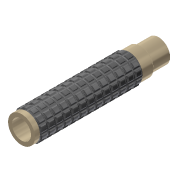
# Autodesk Inventor part: PP-10
Saved by Autodesk Inventor 2022 (Build 260148000, 148)
## iProperties
Created: 2008-09-23
Part Number: PP-10
Document SubType Name: Modeling
Designer: Mark Flayler
Mass: 8.28114 g
Surface Area: 19.0738 cm^2
Volume: 1.05358 cm^3
Density: 7.86 g/cm^3
Material: Steel, Mild
Description: GRIP
Appearance: Titanium - Polished
Author: Mark Flayler
Autodesk Inventor part; units mm, degrees
ref_plane "XZ Plane" through (0, 0, 0) normal (0, 1, 0) x (-1, 0, 0)
sketch "Sketch1" plane through (0, 0, 0) normal (0, 0, 1) x (1, 0, 0)
  line L0 (0, 0) -> (0, 40.8)
  line L1 (2.85, 0) -> (4, 0)
  line L2 (4, 0) -> (4, 35.25)
  line L3 (4, 35.25) -> (3.45, 35.8)
  line L4 (3.45, 35.8) -> (3.45, 40.8)
  line L5 (3.45, 40.8) -> (2.85, 40.8)
  line L6 (2.85, 40.8) -> (2.85, 0)
  dimension "d0" = 40.8
  dimension "d1" = 5.7
  dimension "d2" = 6.9
  dimension "d3" = 35.8
  dimension "d4" = 35.25
  dimension "d5" = 8
  constraints: 14 end point, 3 parallel, 2 horizontal alignment, 2 perpendicular, 1 vertical
  measures "d0" distance of L0.start L0.end
  measures "d1" diameter of L6 L0
  measures "d2" diameter of L4 L0
  measures "d3" vertical distance of L3.end L0.start
  measures "d4" vertical distance of L2.end L0.start
  measures "d5" diameter of L2 L0
revolve "Revolution1" add sketch "Sketch1" angle 360 about axis through (0, 0, 0) along (0, 1, 0)
ref_plane "Work Plane2" through (4.66, 0, 0) normal (1, 0, 0) x (0, 1, 0)
ref_plane "Work Plane4" through (4.035678, 0, 2.33) normal (0.8660254, 0, 0.5) x (0, 1, 0)
ref_plane "Work Plane3" through (0, 0, 0) normal (0.8660254, 0, 0.5) x (0, 1, 0)
sketch "Sketch3" plane through (0, 0, 0) normal (0, 0, 1) x (1, 0, 0)
  line L0 (4.66, 48.96) -> (4.66, -8.16)
  line L1 (-4, 0) -> (4, 0)
  line L2 (0, -8.16) -> (0, 48.96)
  line L3 (4.3, 3.345025) -> (4.3, 2.004975)
  line L4 (4, 35.25) -> (4, 0)
  arc A0 (4.3, 2.004975) -> (4, 1.5) centre (4.575, 1.5) ccw
  arc A1 (4, 3.85) -> (4.3, 3.345025) centre (4.575, 3.85) ccw
  dimension "d11" = 8.6
  dimension "d13" = 1.15
  dimension "d21" = 1.5
  dimension "d22" = 2.35
  constraints: 4 point on circle, 2 centre point, 2 end point, 2 point on line, 2 tangent, 1 equal radius, 1 parallel
  measures "d11" diameter of L3 L2
  measures "d13" diameter of A0
  measures "d21" vertical distance of A0.centre L4.end
  measures "d22" distance of A1.centre A0.centre
revolve "Revolution2" add sketch "Sketch3" angle 360 about axis through (0, 0, 0) along (0, 1, 0)
sketch "Sketch5" plane through (0, 0, 0) normal (0, -1, 0) x (1, 0, 0)
  circle A0 centre (0, 0) radius 2.85
  circle A1 centre (0, 0) radius 4
  circle A2 centre (4.035678, 2.33) radius 0.66
  line L0 (0, 0) -> (4.035678, 2.33) construction
  line L1 (0, 0) -> (1.003206, 0) construction
  line L2 (0.176023, 9.015119) -> (8.069253, -4.656356)
  dimension "d23" = 30
  constraints: 4 end point, 1 centre point, 1 horizontal, 1 point on line, 1 tangent
  measures "d23" angle of L0 L1
extrude "Extrusion1" cut sketch "Sketch5" against normal blind 3.85 contours A2 L2 | A2 L2
pattern_circular "Circular Pattern1" count 12 over 360 about axis through (0, 20.4, 0) along (0, -1, 0) of "Extrusion1"
pattern_linear "Rectangular Pattern1" count 13 spacing 2.35 along (0, 1, 0) of "Extrusion1", "Circular Pattern1", "Revolution2"
body "Solid1"
